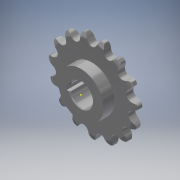
# Autodesk Inventor part: fc17-011
Saved by Autodesk Inventor 2017.1 (Build 211199000, 199)
## iProperties
Created: 2016-12-15
Part Number: fc17-011
Material: Steel
Document SubType Name: Modeling
Designer: PhillipD
Density: 1 g/cm^3
Appearance: Steel
CustomPartVersion: 1
Author: PhillipD
Autodesk Inventor part; units mm, degrees
ref_plane "YZ Plane" through (0, 0, 0) normal (1, 0, 0) x (0, 1, 0)
sketch "Theoretical Tooth Profile" plane through (0, 0, 0) normal (0, 0, 1) x (1, 0, 0)
  circle A0 centre (0, 0) radius 22.9064 construction
  line L0 (0, 0) -> (0, 22.9064) construction
  line L1 (0, 0) -> (9.3169, 20.926) construction
  circle A1 centre (0, 0) radius 25.2633
  arc A2 (-2.0134, 21.2759) -> (2.0134, 21.2759) centre (0, 22.9064) ccw
  line L2 (0, 22.9064) -> (9.3169, 20.926) construction
  line L3 (0, 22.9064) -> (3.1583, 25.4639) construction
  line L4 (3.1583, 25.4639) -> (-2.886, 22.6796) construction
  arc A3 (4.4991, 24.8595) -> (3.1228, 23.1937) centre (6.9566, 21.4277) ccw
  arc A4 (-3.1228, 23.1937) -> (-4.4991, 24.8595) centre (-6.9566, 21.4277) ccw
  line L5 (-6.9566, 21.4277) -> (-3.1228, 23.1937) construction
  arc A5 (-2.886, 22.6796) -> (-2.0134, 21.2759) centre (3.1583, 25.4639) ccw
  line L6 (-2.886, 22.6796) -> (-3.1228, 23.1937)
  arc A6 (2.0134, 21.2759) -> (2.886, 22.6796) centre (-3.1583, 25.4639) ccw
  line L7 (3.1228, 23.1937) -> (2.886, 22.6796)
  line L8 (0, 0) -> (5.2525, 24.7112) construction
  point P0 (4.6584, 21.9162)
  dimension "d0" = 45.8127
  dimension "d2" = 24
  dimension "d3" = 2.5908
  dimension "d10" = 129
  dimension "d11" = 14.267
  dimension "d12" = 4.064
  dimension "d13" = 6.6548
  dimension "d14" = 7.112
  dimension "d23" = 2.8575
  constraints: 18 end point, 15 point on circle, 7 centre point, 3 coincident, 3 point on line, 3 symmetric about line, 3 tangent, 1 equal radius, 1 midpoint, 1 parallel, 1 vertical, 1 other
  measures "d0" diameter of A0
  measures "d2" angle of L1 L0
  measures "d3" radius of A2
  measures "d10" angle of L3 L0
  measures "d11" angle of L4 L3
  measures "d12" distance of L2.start L3.end
  measures "d13" distance of L3.end L4.end
  measures "d14" distance of A3.centre L0.end
  measures "d23" distance from line of L8.end L2
sketch "Tooth Profile" plane through (0, 0, 0) normal (0, 0, 1) x (1, 0, 0)
  circle A0 centre (0, 0) radius 25.2633 projected
  line L0 (0, 0) -> (0, 22.9064) construction
  line L1 (0, 22.9064) -> (2.3848, 21.8941) construction
  arc A1 (-2.3848, 21.8941) -> (2.3848, 21.8941) centre (0, 22.9064) ccw
  line L2 (-2.3848, 21.8941) -> (0, 22.9064) construction
  arc A2 (-2.3848, 21.8941) -> (-4.3245, 24.8904) centre (-11.9242, 17.8448) ccw
  arc A3 (4.3245, 24.8904) -> (2.3848, 21.8941) centre (11.9242, 17.8448) ccw
  dimension "d44" = 134
  dimension "d45" = 2.5908
  dimension "d46" = 10.3632
  constraints: 8 point on circle, 7 end point, 3 centre point, 2 tangent, 1 coincident, 1 equal radius, 1 symmetric about line, 1 vertical
  measures "d44" angle of L1 L2
  measures "d45" radius of A1
  measures "d46" radius of A3
sketch "Section Profile" plane through (0, 0, 0) normal (1, 0, 0) x (0, 1, 0)
  line L0 (25.2633, 0) -> (-25.2633, 0) projected
  line L1 (16.8813, 2.2967) -> (-16.8813, 2.2967)
  line L2 (-16.8813, 2.2967) -> (-16.8813, -2.2967)
  line L3 (-16.8813, -2.2967) -> (16.8813, -2.2967)
  line L4 (16.8813, -2.2967) -> (16.8813, 2.2967)
  line L5 (16.8813, 2.2967) -> (25.2633, 2.2967) construction
  line L6 (25.2633, 2.2967) -> (25.2633, -2.2967) construction
  line L7 (25.2633, -2.2967) -> (16.8813, -2.2967) construction
  line L8 (16.8813, -2.2967) -> (16.8813, 2.2967)
  arc A0 (25.2633, 1.106) -> (20.4996, 2.2967) centre (20.4996, -7.8284) ccw
  arc A1 (20.4996, -2.2967) -> (25.2633, -1.106) centre (20.4996, 7.8284) ccw
  line L9 (20.4996, 2.2967) -> (0, 2.2967)
  line L10 (0, 2.2967) -> (0, -2.2967)
  line L11 (0, -2.2967) -> (20.4996, -2.2967)
  line L12 (0, 2.2967) -> (0, -2.2967)
  line L13 (25.2633, 1.106) -> (25.2633, -1.106)
  point P0 (0, 0)
  point P1 (0, 0)
  dimension "d30" = 4.5933
  dimension "d31" = 33.7626
  dimension "d32" = 4.5933
  dimension "d33" = 1.1906
  dimension "d34" = 10.1251
  dimension "d43" = 2.2967
  constraints: 26 end point, 7 midpoint, 5 perpendicular, 4 parallel, 4 point on circle, 3 point on line, 3 symmetric about line, 2 centre point, 2 horizontal, 2 tangent, 1 collinear, 1 other
  measures "d30" distance between parallel lines of L7 L5
  measures "d31" distance between parallel lines of L2 L4
  measures "d32" distance between parallel lines of L3 L1
  measures "d33" distance from line of L13.start L5
  measures "d34" radius of A0
  measures "d43" distance between parallel lines of L3 L0
revolve "Shroud" add sketch "Section Profile" angle 360 about axis through (0, 0, 2.2967) along (0, 0, -1) contours L10 L3 L2 L0 | L0 L2 L1 L10
revolve "Strand" add sketch "Section Profile" angle 360 about axis through (0, 0, 2.2967) along (0, 0, -1) contours L13 A1 L11 L4 L0 | L0 L4 L9 A0 L13 | L4 L3 L10 L0 | L0 L10 L1 L4
pattern_of_one "Strand Pattern"
extrude "Theoretical Tooth" cut sketch "Theoretical Tooth Profile" along normal through all both and the other way through all contours A3 L7 A6 A2 A5 L6 A4 A1 picked at (-0.5023, 22.59)
extrude "Tooth" [suppressed]
pattern_circular "Tooth Pattern" count 15 over 360 about axis through (0, 0, -10) along (0, 0, 1) of "Theoretical Tooth"
ref_plane "Timing Plane" through (0, 22.9064, 0) normal (1, 0, 0) x (0, 1, 0)
ref_plane "Work Plane3" through (0, 22.9064, 0) normal (0, 0, 1) x (1, 0, 0)
sketch "Sketch4" plane through (0, 0, 0) normal (0, 1, 0) x (-1, 0, 0)
  line L0 (30.7785, 2.032) -> (-28.6751, 2.032)
  line L1 (-28.6751, 2.032) -> (-28.6751, -2.032)
  line L2 (-28.6751, -2.032) -> (30.7785, -2.032)
  line L3 (30.7785, -2.032) -> (30.7785, 2.032)
  line L4 (-42.2709, 0) -> (44.3743, 0) projected
  line L5 (31.9964, -3.2499) -> (-29.893, -3.2499)
  line L6 (-29.893, -3.2499) -> (-29.893, 3.2499)
  line L7 (-29.893, 3.2499) -> (31.9964, 3.2499)
  line L8 (31.9964, 3.2499) -> (31.9964, -3.2499)
  point P0 (0, 0)
  dimension "d51" = 4.064
  dimension "d52" = 2.032
  constraints: 16 end point, 4 parallel, 2 perpendicular, 1 horizontal, 3 other
  measures "d51" distance of L2.end L0.start
  measures "d52" distance between parallel lines of L4 L0
extrude "Extrusion4" cut sketch "Sketch4" along normal mid plane 69.65 contours L0 L1 L4 L6 L7 L8 L3 | L4 L8 L5 L6 L1 L2 L3
sketch "Sketch5" plane through (0, 22.9064, 2.032) normal (0, 0, 1) x (1, 0, 0)
  circle A0 centre (0, -22.9064) radius 6.3754
  circle A1 centre (0, -22.9064) radius 12.7
  point P0 (0, -22.9064)
  dimension "d55" = 12.7508
  dimension "d56" = 25.4
  constraints: 2 centre point, 2 coincident
  measures "d55" diameter of A0
  measures "d56" diameter of A1
extrude "Extrusion5" add sketch "Sketch5" along normal blind 6.223
extrude "Extrusion6" cut sketch "Sketch5" against normal blind 25.777 contours A0
sketch "Sketch6" plane through (0, 0, 8.255) normal (0, 0, 1) x (1, 0, 0)
  point P0 (0, 0)
sketch "Sketch8" plane through (0, 0, 8.255) normal (0, 0, 1) x (1, 0, 0)
  line L0 (-7.9629, 1.5875) -> (-6.1746, 1.5875)
  arc A0 (-6.1746, -1.5875) -> (-6.1746, 1.5875) centre (0, 0) ccw
  line L1 (-6.1746, -1.5875) -> (-7.9629, -1.5875)
  line L2 (-7.9629, 1.5875) -> (-7.9629, -1.5875)
  line L3 (33.2891, 0) -> (-36.5609, 0) construction
  line L4 (0, -16.6765) -> (0, 37.2985) construction
  circle A1 centre (0, 0) radius 6.3754 projected
  dimension "d66" = 6.3754
  dimension "d67" = 3.175
  dimension "d68" = 7.9629
  constraints: 10 end point, 2 parallel, 2 point on circle, 2 point on line, 1 centre point, 1 coincident, 1 horizontal, 1 vertical, 1 other
  measures "d66" radius of A0
  measures "d67" distance between parallel lines of L0 L1
  measures "d68" distance from line of L2 A0.centre
extrude "Key Square (Hole)1" cut sketch "Sketch8" against normal up to next
chamfer "Chamfer1" distance 0.508 angle 45 2 edges at (6.3754, 0, 8.255) (6.3754, 0, -2.032)
equation "\"d3\" = 0.5 * da_Dr + da_SC"
equation "\"d12\" = 0.8 * da_Dr"
equation "\"d13\" = 1.3 * da_Dr + da_SC"
equation "\"d14\" = 1.4 * da_Dr"
equation "\"d23\" = da_Ha"
equation "\"d44\" = da_Alfa"
equation "\"d45\" = da_Ri"
equation "\"d46\" = da_Re"
equation "\"d30\" = da_Bf"
equation "\"d31\" = da_Ds"
equation "\"d32\" = da_Bs"
equation "\"d33\" = da_Ba"
equation "\"d34\" = da_Rx"
equation "\"d40\" = da_pt"
equation "\"form_type\" = 0"
equation "\"d52\" = 0.5 * d51"
equation "\"da_p\" = 9.525"
equation "\"da_Dr\" = 5.08"
equation "\"da_SC\" = 0.0508"
equation "\"da_Ha\" = 2.8575"
equation "\"da_pt\" = 10.1346"
equation "\"da_Bf\" = 4.59334"
equation "\"da_Ba\" = 1.19063"
equation "\"da_Rx\" = 10.12508"
equation "\"da_Ra\" = 0.381"
equation "\"da_Bs\" = 4.59334"
equation "\"da_Ds\" = 33.7626"
equation "\"da_Re\" = 10.3632"
equation "\"da_Ri\" = 2.5908"
equation "\"da_Alfa\" = 134deg"
body "Solid1"
